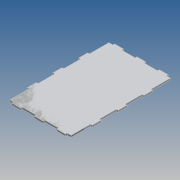
# Autodesk Inventor part: BaseSupportBatterie1
Saved by Autodesk Inventor 2019 (Build 230136000, 136)
## iProperties
Created: 2019-08-27
Part Number: BaseSupportBatterie1
Material: PVC-U
Document SubType Name: Modeling
Designer: jeremias.salamin
Density: 1.4 g/cm^3
Appearance: Lisse - Blanc
Description: SupportBatterie1
Mass: 10.0558 g
Surface Area: 94.2192 cm^2
Volume: 7.18272 cm^3
Author: jeremias.salamin
Autodesk Inventor part; units mm, degrees
ref_plane "YZ Plane" through (0, 0, 0) normal (1, 0, 0) x (0, 1, 0)
ref_plane "XZ Plane" through (0, 0, 0) normal (0, 1, 0) x (-1, 0, 0)
ref_plane "XY Plane" through (0, 0, 0) normal (0, 0, 1) x (1, 0, 0)
sketch "Sketch1" plane through (0, 0, 0) normal (0, 0, 1) x (1, 0, 0)
  line L0 (0, 62.09) -> (0, -62.09) construction
  line L1 (-38.5, 0) -> (38.5, 0) construction
  line L2 (27.5, -44.35) -> (-27.5, -44.35)
  line L3 (-27.5, -44.35) -> (-27.5, 44.35)
  line L4 (-27.5, 44.35) -> (27.5, 44.35)
  line L5 (27.5, 44.35) -> (27.5, -44.35)
  line L6 (27.5, -44.35) -> (-27.5, 44.35) construction
  line L7 (-27.5, -44.35) -> (27.5, 44.35) construction
  point P0 (0, 0)
  dimension "d0" = 55
  dimension "d1" = 88.7
  constraints: 12 end point, 2 midpoint, 2 parallel, 1 horizontal, 1 perpendicular
  measures "d0" distance of L3.end L4.end
  measures "d1" distance of L2.end L3.end
extrude "Extrusion1" add sketch "Sketch1" along normal mid plane 1.6
sketch "Esquisse2" plane through (0, 0, 0.8) normal (0, 0, 1) x (1, 0, 0)
  line L0 (-27.5, -44.35) -> (27.5, -44.35) construction
  line L1 (27.5, -44.35) -> (27.5, 44.35) construction
  line L2 (27.5, 44.35) -> (-27.5, 44.35) construction
  line L3 (-27.5, 44.35) -> (-27.5, -44.35) construction
  line L4 (0, 62.09) -> (0, -62.09) construction
  line L5 (-40.42, 0) -> (38.82, 0) construction
  line L6 (-27.5, -27) -> (-29.1, -27)
  line L7 (-29.1, -27) -> (-29.1, -19)
  line L8 (-29.1, -19) -> (-27.5, -19)
  line L9 (-27.5, -19) -> (-27.5, -27)
  line L10 (-27.5, -4) -> (-29.1, -4)
  line L11 (-29.1, -4) -> (-29.1, 4)
  line L12 (-29.1, 4) -> (-27.5, 4)
  line L13 (-27.5, 4) -> (-27.5, -4)
  line L14 (-27.5, 19) -> (-29.1, 19)
  line L15 (-29.1, 19) -> (-29.1, 27)
  line L16 (-29.1, 27) -> (-27.5, 27)
  line L17 (-27.5, 27) -> (-27.5, 19)
  point P0 (0, 0)
  dimension "d4" = 1.6
  dimension "d5" = 8
  dimension "d8" = 23
  constraints: 24 end point, 2 parallel, 1 horizontal, 1 perpendicular, 1 point on line, 1 vertical, 17 other
  measures "d4" distance of L7.end L8.end
  measures "d5" distance of L6.end L7.end
  measures "d8" distance of L6.start L10.start
extrude "Extrusion2" add sketch "Esquisse2" against normal blind 1.6
mirror "Symétrie1" about plane through (0, 0, 0) normal (1, 0, 0) of "Extrusion2"
sketch "Esquisse3" plane through (0, 0, 0.8) normal (0, 0, 1) x (1, 0, 0)
  line L0 (-29.1, 27) -> (-27.5, 27) construction
  line L1 (-27.5, 27) -> (-27.5, 44.35) construction
  line L2 (-27.5, 44.35) -> (27.5, 44.35) construction
  line L3 (27.5, 44.35) -> (27.5, 27) construction
  line L4 (27.5, 27) -> (29.1, 27) construction
  line L5 (29.1, 27) -> (29.1, 19) construction
  line L6 (29.1, 19) -> (27.5, 19) construction
  line L7 (27.5, 19) -> (27.5, 4) construction
  line L8 (27.5, 4) -> (29.1, 4) construction
  line L9 (29.1, 4) -> (29.1, -4) construction
  line L10 (29.1, -4) -> (27.5, -4) construction
  line L11 (27.5, -4) -> (27.5, -19) construction
  line L12 (27.5, -19) -> (29.1, -19) construction
  line L13 (29.1, -19) -> (29.1, -27) construction
  line L14 (29.1, -27) -> (27.5, -27) construction
  line L15 (27.5, -27) -> (27.5, -44.35) construction
  line L16 (27.5, -44.35) -> (-27.5, -44.35) construction
  line L17 (-27.5, -44.35) -> (-27.5, -27) construction
  line L18 (-27.5, -27) -> (-29.1, -27) construction
  line L19 (-29.1, -27) -> (-29.1, -19) construction
  line L20 (-29.1, -19) -> (-27.5, -19) construction
  line L21 (-27.5, -19) -> (-27.5, -4) construction
  line L22 (-27.5, -4) -> (-29.1, -4) construction
  line L23 (-29.1, -4) -> (-29.1, 4) construction
  line L24 (-29.1, 4) -> (-27.5, 4) construction
  line L25 (-27.5, 4) -> (-27.5, 19) construction
  line L26 (-27.5, 19) -> (-29.1, 19) construction
  line L27 (-29.1, 19) -> (-29.1, 27) construction
  line L28 (0, 62.09) -> (0, -62.09) construction
  line L29 (-40.74, 0) -> (40.74, 0) construction
  line L30 (-27.5, -44.35) -> (27.5, -44.35) construction
  line L31 (27.5, -44.35) -> (27.5, -27) construction
  line L32 (27.5, -27) -> (29.1, -27) construction
  line L33 (29.1, -27) -> (29.1, -19) construction
  line L34 (29.1, -19) -> (27.5, -19) construction
  line L35 (27.5, -19) -> (27.5, -4) construction
  line L36 (27.5, -4) -> (29.1, -4) construction
  line L37 (29.1, -4) -> (29.1, 4) construction
  line L38 (29.1, 4) -> (27.5, 4) construction
  line L39 (27.5, 4) -> (27.5, 19) construction
  line L40 (27.5, 19) -> (29.1, 19) construction
  line L41 (29.1, 19) -> (29.1, 27) construction
  line L42 (29.1, 27) -> (27.5, 27) construction
  line L43 (27.5, 27) -> (27.5, 44.35) construction
  line L44 (27.5, 44.35) -> (-27.5, 44.35) construction
  line L45 (-27.5, 44.35) -> (-27.5, 27) construction
  line L46 (-29.1, 27) -> (-27.5, 27) construction
  line L47 (-29.1, 19) -> (-29.1, 27) construction
  line L48 (-27.5, 19) -> (-29.1, 19) construction
  line L49 (-27.5, 19) -> (-27.5, 4) construction
  line L50 (-29.1, 4) -> (-27.5, 4) construction
  line L51 (-29.1, -4) -> (-29.1, 4) construction
  line L52 (-27.5, -4) -> (-29.1, -4) construction
  line L53 (-27.5, -4) -> (-27.5, -19) construction
  line L54 (-29.1, -19) -> (-27.5, -19) construction
  line L55 (-29.1, -27) -> (-29.1, -19) construction
  line L56 (-27.5, -27) -> (-29.1, -27) construction
  line L57 (-27.5, -27) -> (-27.5, -44.35) construction
  line L58 (24, 44.35) -> (16, 44.35)
  line L59 (16, 44.35) -> (16, 45.95)
  line L60 (16, 45.95) -> (24, 45.95)
  line L61 (24, 45.95) -> (24, 44.35)
  line L62 (4, 44.35) -> (-4, 44.35)
  line L63 (-4, 45.95) -> (4, 45.95)
  line L64 (4, 45.95) -> (4, 44.35)
  line L65 (-4, 44.35) -> (-4, 45.95)
  line L66 (-16, 44.35) -> (-24, 44.35)
  line L67 (-24, 45.95) -> (-16, 45.95)
  line L68 (-16, 45.95) -> (-16, 44.35)
  line L69 (-24, 44.35) -> (-24, 45.95)
  point P0 (0, 0)
  dimension "d15" = 8
  dimension "d16" = 1.6
  dimension "d19" = 20
  constraints: 24 end point, 2 horizontal, 2 parallel, 1 perpendicular, 1 point on line, 17 other
  measures "d15" distance of L59.end L60.end
  measures "d16" distance of L58.end L59.end
  measures "d19" distance of L58.start L62.start
extrude "Extrusion3" add sketch "Esquisse3" against normal blind 1.6
mirror "Symétrie2" about plane through (0, 0, 0) normal (0, 1, 0) of "Extrusion3"
sketch "Esquisse4" plane through (-29.1, -4, 0.8) normal (-1, 0, 0) x (0, 0, 1)
  point P0 (-0.8, 4)
sketch "Esquisse5" plane through (0, 0, 0.8) normal (0, 0, 1) x (1, 0, 0)
  line L0 (-27.5, 31) -> (-29.1, 31)
  line L1 (-29.1, 31) -> (-29.1, 2)
  line L2 (-29.1, 2) -> (-27.5, 2)
  line L3 (-27.5, 2) -> (-27.5, -2)
  line L4 (-27.5, -2) -> (-29.1, -2)
  line L5 (-29.1, -2) -> (-29.1, -31)
  line L6 (-29.1, -31) -> (-27.5, -31)
  line L7 (-27.5, -31) -> (-27.5, -39)
  line L8 (-27.5, -39) -> (-29.1, -39)
  line L9 (-29.1, -39) -> (-29.1, -44.35)
  line L10 (-29.1, -44.35) -> (-32.6, -44.35)
  line L11 (-32.6, -44.35) -> (-32.6, -45.95)
  line L12 (-32.6, -45.95) -> (-40.6, -45.95)
  line L13 (-40.6, -45.95) -> (-40.6, -44.35)
  line L14 (-40.6, -44.35) -> (-44.1, -44.35)
  line L15 (-44.1, -44.35) -> (-44.1, 44.35)
  line L16 (-44.1, 44.35) -> (-29.1, 44.35)
  line L17 (-29.1, 44.35) -> (-29.1, 39)
  line L18 (-29.1, 39) -> (-27.5, 39)
  line L19 (-27.5, 39) -> (-27.5, 31)
  point P0 (0, 0)
  constraints: 40 end point, 10 horizontal, 10 vertical, 20 other
extrude "Extrusion4" cut sketch "Esquisse5" against normal blind 1.6
